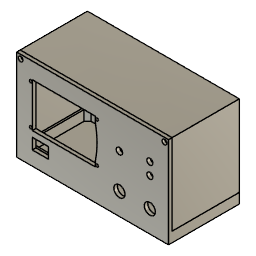
Andrew Block 1 v1 v24 (Autodesk Fusion 360 design; units mm, degrees)
Autodesk Fusion 360 part; units mm, degrees
sketch "Sketch1" plane through (0, 0, 0) normal (0, 0, 1) x (1, 0, 0)
  line L0 (0, 0) -> (190.5, 0)
  line L1 (190.5, 0) -> (190.5, 88.9)
  line L2 (190.5, 88.9) -> (0, 88.9)
  line L3 (0, 88.9) -> (0, 0)
  constraint horizontal L0
  constraint vertical L1
  constraint horizontal L2
  constraint vertical L3
  constraint coincident L0.start L3.end
extrude "Extrude1" add sketch "Sketch1" along normal blind 114.3 makes body 1
ref_plane "WorkPlane1" through (0, 0, 12.7) normal (0, 0, 1) x (1, 0, 0)
shell "Shell1" thickness 4.445 removed faces 0 bodies 1
chamfer "Chamfer4" distance 6.35 angle 45 4 edges at (4.445, 84.455, 57.15) (186.055, 84.455, 57.15) (4.445, 4.445, 57.15) (186.055, 4.445, 57.15) on bodies 1
split "Split1" by plane through (0, 0, 12.7) normal (0, 0, 1) bodies 1 makes body 2 at (127, 88.9, 46.5667)
chamfer "Chamfer5" distance 6.35 angle 45 4 edges at (4.445, 44.45, 109.855) (95.25, 84.455, 109.855) (95.25, 4.445, 109.855) (186.055, 44.45, 109.855) on bodies 2
sketch "Sketch2" plane through (0, 0, 4.445) normal (0, 0, 1) x (-1, 0, 0)
  line L0 (-4.445, -78.105) -> (-4.445, -10.795)
  line L1 (-10.795, -4.445) -> (-179.705, -4.445)
  line L2 (-186.055, -10.795) -> (-186.055, -78.105)
  line L3 (-179.705, -84.455) -> (-10.795, -84.455)
  line L4 (-7.62, -81.28) -> (-182.88, -81.28)
  line L5 (-182.88, -81.28) -> (-182.88, -7.62)
  line L6 (-182.88, -7.62) -> (-7.62, -7.62)
  line L7 (-7.62, -7.62) -> (-7.62, -81.28)
  line L8 (-182.88, -81.28) -> (-184.658, -83.058) construction
  line L9 (-182.88, -81.28) -> (-180.3655, -81.28) construction
  line L10 (-7.62, -7.62) -> (-5.8419, -5.8419) construction
  line L11 (-7.62, -7.62) -> (-5.1054, -7.62) construction
  line L12 (-184.658, -83.058) -> (-5.8419, -83.058)
  line L13 (-5.8419, -83.058) -> (-5.8419, -5.8419)
  line L14 (-5.8419, -5.8419) -> (-184.658, -5.8419)
  line L15 (-184.658, -5.8419) -> (-184.658, -83.058)
  line L16 (-179.705, -4.445) -> (-186.055, -10.795)
  line L17 (-186.055, -78.105) -> (-179.705, -84.455)
  line L18 (-10.795, -84.455) -> (-4.445, -78.105)
  line L19 (-4.445, -10.795) -> (-10.795, -4.445)
  dimension "d7" = 135
  dimension "d8" = 45
  dimension "d9" = 2.5146
  constraint horizontal L4
  constraint vertical L5
  constraint horizontal L6
  constraint vertical L7
  constraint horizontal L9
  constraint horizontal L11
  constraint horizontal L12
  constraint vertical L13
  constraint horizontal L14
  constraint vertical L15
  measures "d7" angle of L8 L9
  measures "d8" angle of L10 L11
  measures "d9" distance of L6.end L10.end
sketch "Sketch6" plane through (0, 0, 0) normal (0, 0, -1) x (1, 0, 0)
  line L0 (0, 0) -> (0, -88.9)
  line L1 (0, -88.9) -> (190.5, -88.9)
  line L2 (190.5, -88.9) -> (190.5, 0)
  line L3 (190.5, 0) -> (0, 0)
  line L4 (5.08, -83.82) -> (185.42, -83.82)
  line L5 (185.42, -83.82) -> (185.42, -5.08)
  line L6 (185.42, -5.08) -> (5.08, -5.08)
  line L7 (5.08, -5.08) -> (5.08, -83.82)
  dimension "d42" = -5.08
sketch "Sketch8" plane through (0, 0, 0) normal (0, -1, 0) x (1, 0, 0)
  line L0 (0, 12.7) -> (190.5, 12.7)
  line L1 (190.5, 12.7) -> (190.5, 114.3)
  line L2 (190.5, 114.3) -> (0, 114.3)
  line L3 (0, 114.3) -> (0, 12.7)
  line L4 (5.08, 17.78) -> (185.42, 17.78)
  line L5 (185.42, 17.78) -> (185.42, 109.22)
  line L6 (185.42, 109.22) -> (5.08, 109.22)
  line L7 (5.08, 109.22) -> (5.08, 17.78)
  dimension "d76" = -5.08
hole "Hole4" at (5.08, 0, 109.22) at (185.42, 0, 109.22) direction (0, 1, 0) diameter 2.54 depth 25.4 tip angle 118 counterbore diameter 5.969 counterbore depth 3.3528 bodies 2
hole "Hole2" at (5.08, 83.82, 0) at (185.42, 83.82, 0) direction (0, 0, 1) diameter 4.318 depth 19.7 tip angle 180 bodies 2
hole "Hole1" at (5.08, 83.82, 0) at (185.42, 83.82, 0) direction (0, 0, 1) diameter 3.556 depth 254 tip angle 118 counterbore diameter 5.969 counterbore depth 3.3528 bodies 1
sketch "Sketch5" plane through (0, 0, 4.445) normal (0, 0, 1) x (-1, 0, 0)
  line L0 (-4.445, -78.105) -> (-4.445, -10.795)
  line L1 (-10.795, -4.445) -> (-179.705, -4.445)
  line L2 (-186.055, -10.795) -> (-186.055, -78.105)
  line L3 (-179.705, -84.455) -> (-10.795, -84.455)
  line L4 (-179.705, -4.445) -> (-186.055, -10.795)
  line L5 (-186.055, -78.105) -> (-179.705, -84.455)
  line L6 (-10.795, -84.455) -> (-4.445, -78.105)
  line L7 (-4.445, -10.795) -> (-10.795, -4.445)
  line L8 (-178.3796, -81.2552) -> (-12.1204, -81.2552)
  line L9 (-12.1204, -81.2552) -> (-7.6448, -76.7796)
  line L10 (-7.6448, -76.7796) -> (-7.6448, -12.1204)
  line L11 (-7.6448, -12.1204) -> (-12.1204, -7.6448)
  line L12 (-12.1204, -7.6448) -> (-178.3796, -7.6448)
  line L13 (-178.3796, -7.6448) -> (-182.8552, -12.1204)
  line L14 (-182.8552, -12.1204) -> (-182.8552, -76.7796)
  line L15 (-182.8552, -76.7796) -> (-178.3796, -81.2552)
  line L16 (-179.3799, -83.6701) -> (-11.1201, -83.6701)
  line L17 (-11.1201, -83.6701) -> (-5.2299, -77.7799)
  line L18 (-5.2299, -77.7799) -> (-5.2299, -11.1201)
  line L19 (-5.2299, -11.1201) -> (-11.1201, -5.2299)
  line L20 (-11.1201, -5.2299) -> (-179.3799, -5.2299)
  line L21 (-179.3799, -5.2299) -> (-185.2701, -11.1201)
  line L22 (-185.2701, -11.1201) -> (-185.2701, -77.7799)
  line L23 (-185.2701, -77.7799) -> (-179.3799, -83.6701)
  dimension "d35" = -3.1998
  dimension "d36" = -0.7849
extrude "Extrude6" add sketch "Sketch5" along normal blind 12.7 contours L16 L17 L18 L19 L20 L21 L22 L23 bodies 1
extrude "Extrude7" add 1 faces at (67.2067, 84.1934, 4.445) along direction (0, 0, 1) blind 5.08 on bodies 1 bodies 1
sketch "Sketch4" plane through (0, 0, 0) normal (0, -1, 0) x (1, 0, 0)
  line L0 (0, 12.7) -> (190.5, 12.7)
  line L1 (190.5, 12.7) -> (190.5, 114.3)
  line L2 (190.5, 114.3) -> (0, 114.3)
  line L3 (0, 114.3) -> (0, 12.7)
  circle A0 centre (128.9671, 27.5835) radius 7
  circle A1 centre (167.0671, 27.5835) radius 7
  circle A2 centre (5.08, 109.22) radius 2.9845
  circle A3 centre (185.42, 109.22) radius 2.9845
  circle A4 centre (167.0671, 78.74) radius 3.81
  circle A5 centre (167.0671, 63.5) radius 3.81
  line L4 (167.0671, 27.5835) -> (167.0671, 63.5) construction
  line L5 (128.9671, 27.5835) -> (128.9671, 63.5) construction
  line L6 (19.812, 17.78) -> (39.878, 17.78)
  line L7 (39.878, 17.78) -> (39.878, 31.496)
  line L8 (19.812, 31.496) -> (19.812, 17.78)
  circle A6 centre (128.9022, 71.12) radius 4.064
  line L9 (15.24, 93.98) -> (103.378, 93.98)
  line L10 (103.378, 93.98) -> (103.378, 38.862)
  line L11 (103.378, 38.862) -> (15.24, 38.862)
  line L12 (15.24, 38.862) -> (15.24, 93.98)
  line L13 (15.24, 93.98) -> (19.812, 93.98)
  line L14 (103.378, 93.98) -> (98.806, 93.98)
  line L15 (19.812, 93.98) -> (19.812, 38.862)
  line L16 (98.806, 93.98) -> (98.806, 38.862)
  line L17 (17.78, 91.44) -> (100.838, 91.44) construction
  line L18 (100.838, 91.44) -> (100.838, 41.402) construction
  line L19 (100.838, 41.402) -> (17.78, 41.402) construction
  line L20 (17.78, 41.402) -> (17.78, 91.44) construction
  line L21 (98.806, 86.4684) -> (100.838, 86.4684)
  line L22 (100.838, 86.4684) -> (100.838, 45.589)
  line L23 (100.838, 45.589) -> (98.806, 45.589)
  line L24 (98.806, 45.589) -> (98.806, 86.4684)
  line L25 (19.812, 31.496) -> (39.878, 31.496)
  line L26 (19.812, 48.3189) -> (19.812, 17.78) construction
  point P0 (128.9671, 63.5)
  dimension "d62" = 14
  dimension "d63" = 14
  dimension "d94" = 7.62
  dimension "d95" = 7.62
  dimension "d103" = 20.066
  dimension "d104" = 13.716
  dimension "d111" = 8.128
  dimension "d114" = 88.138
  dimension "d115" = 55.118
  dimension "d116" = 4.572
  dimension "d117" = 4.572
  dimension "d118" = 2.54
  constraint coincident A1.centre L4.start
  constraint vertical L4
  constraint coincident A0.centre L5.start
  constraint perpendicular L0 L5
  constraint horizontal L6
  constraint vertical L7
  constraint vertical L8
  constraint horizontal L9
  constraint vertical L10
  constraint horizontal L11
  constraint vertical L12
  constraint perpendicular L10 L14
  constraint coincident L11 L15.end
  constraint perpendicular L11 L15
  constraint coincident L11 L16.end
  constraint perpendicular L11 L16
  constraint horizontal L21
  constraint vertical L22
  constraint horizontal L23
  constraint vertical L24
  constraint coincident L18 L22.end
  constraint coincident L16 L21.start
  constraint perpendicular L7 L25
  constraint coincident L15 L26.start
  constraint perpendicular L11 L26
  measures "d62" diameter of A0
  measures "d63" diameter of A1
  measures "d94" diameter of A4
  measures "d95" diameter of A5
  measures "d103" distance of L6.start L6.end
  measures "d104" distance of L6.start L8.start
  measures "d111" diameter of A6
  measures "d114" distance of L9.start L9.end
  measures "d115" distance of L9.start L11.end
  measures "d116" distance of L9.start L13.end
  measures "d117" distance of L9.end L14.end
hole "Hole3" at (17.78, 0, 91.44) at (17.78, 0, 41.402) at (100.838, 0, 91.44) at (100.838, 0, 41.402) direction (0, 1, 0) diameter 3.5 depth 12.7 tip angle 180 bodies 2
extrude "Extrude8" cut sketch "Sketch4" against normal blind 30.48 contours A0 | A1 | A4 | A5 | L6 L7 L8 L25 | A6 | L9 L11 L15 L16 L24 | L16 L21 L22 L23 L24 bodies 2
sketch "Sketch7" plane through (0, 0, 4.445) normal (0, 0, 1) x (-1, 0, 0)
  line L0 (-178.3796, -81.2552) -> (-12.1204, -81.2552)
  line L1 (-7.6448, -76.7796) -> (-7.6448, -12.1204)
  line L2 (-12.1204, -7.6448) -> (-178.3796, -7.6448)
  line L3 (-182.8552, -12.1204) -> (-182.8552, -76.7796)
  line L4 (-76.4252, -76.6519) -> (-76.4252, -12.2481) construction
  circle A0 centre (-76.4252, -76.6519) radius 4.6032
  circle A1 centre (-76.4252, -76.6519) radius 2.159
  circle A2 centre (-76.4252, -12.2481) radius 2.159
  circle A3 centre (-76.4252, -12.2481) radius 4.6032
  line L5 (-12.1204, -81.2552) -> (-7.6448, -76.7796)
  line L6 (-7.6448, -12.1204) -> (-12.1204, -7.6448)
  line L7 (-178.3796, -7.6448) -> (-182.8552, -12.1204)
  line L8 (-182.8552, -76.7796) -> (-178.3796, -81.2552)
  line L9 (-14.0271, -12.2481) -> (-176.4729, -12.2481) construction
  line L10 (-176.4729, -12.2481) -> (-178.2519, -14.0271)
  line L11 (-178.2519, -14.0271) -> (-178.2519, -74.8729) construction
  line L12 (-178.2519, -74.8729) -> (-176.4729, -76.6519)
  line L13 (-176.4729, -76.6519) -> (-14.0271, -76.6519) construction
  line L14 (-14.0271, -76.6519) -> (-12.2481, -74.8729)
  line L15 (-12.2481, -74.8729) -> (-12.2481, -14.0271) construction
  line L16 (-12.2481, -14.0271) -> (-14.0271, -12.2481)
  line L17 (-162.5137, -12.2481) -> (-162.5137, -76.6519) construction
  circle A4 centre (-162.7852, -12.8831) radius 4.6032
  circle A5 centre (-162.7852, -12.8831) radius 2.159
  circle A6 centre (-162.7852, -76.0169) radius 4.6032
  circle A7 centre (-162.7852, -76.0169) radius 2.159
  dimension "d52" = -4.6032
  dimension "d53" = 4.318
  dimension "d56" = 4.318
  dimension "d71" = 4.318
  dimension "d72" = 4.318
  constraint coincident L4.start L13
  constraint coincident L4.end L9
  constraint perpendicular L4 L9
  constraint coincident L4.start A0.centre
  constraint tangent L0 A0
  constraint concentric A0 A1
  constraint concentric A2 A3
  constraint tangent L2 A3
  constraint coincident L9 L17.start
  constraint coincident L13 L17.end
  constraint perpendicular L13 L17
  constraint concentric A4 A5
  constraint concentric A6 A7
  measures "d53" diameter of A1
  measures "d56" diameter of A2
  measures "d71" diameter of A5
  measures "d72" diameter of A7
ref_plane "WorkPlane2" through (0, 4.445, 0) normal (0, 1, 0) x (0, 0, 1)
chamfer "Chamfer3" distance 1.016 angle 45 1 edges at (187.4329, 84.6007, 12.7) on bodies 2
chamfer "Chamfer3" distance 1.016 angle 45 1 edges at (7.0929, 84.6007, 12.7) on bodies 2
split "Split2" by plane through (0, 4.445, 0) normal (0, 1, 0) bodies 2 makes body 3 at (127, 88.9, 46.5667)
fillet "Fillet1" radius 99.06 2 edges at (100.838, 2.2225, 86.4684) (100.838, 2.2225, 45.589) on bodies 2
combine "Combine1" operation add target body 1 tool bodies 2
hole "Hole5" at (5.08, 0, 109.22) at (185.42, 0, 109.22) direction (0, 1, 0) diameter 4.318 depth 19.7 tip angle 180 bodies 3
sketch "Sketch11" plane through (0, 4.445, 0) normal (0, 1, 0) x (-1, 0, 0)
  circle A0 centre (-167.0671, 27.5835) radius 7
  circle A1 centre (-167.0671, 78.74) radius 3.81
  circle A2 centre (-128.9671, 27.5835) radius 7
  circle A3 centre (-167.0671, 63.5) radius 3.81
  circle A4 centre (-5.08, 109.22) radius 1.27
  circle A5 centre (-185.42, 109.22) radius 1.27
  line L0 (-179.705, 9.525) -> (-10.795, 9.525)
  line L1 (-10.795, 9.525) -> (-10.795, 12.7)
  line L2 (-10.795, 12.7) -> (0, 12.7)
  line L3 (0, 12.7) -> (0, 114.3)
  line L4 (0, 114.3) -> (-190.5, 114.3)
  line L5 (-190.5, 114.3) -> (-190.5, 12.7)
  line L6 (-190.5, 12.7) -> (-179.705, 12.7)
  line L7 (-179.705, 12.7) -> (-179.705, 9.525)
  circle A6 centre (-128.9022, 71.12) radius 4.064
  circle A7 centre (-100.838, 41.402) radius 1.75
  circle A8 centre (-17.78, 41.402) radius 1.75
  circle A9 centre (-17.78, 91.44) radius 1.75
  circle A10 centre (-100.838, 91.44) radius 1.75
  line L8 (-19.812, 38.862) -> (-98.806, 38.862)
  line L9 (-98.806, 38.862) -> (-98.806, 45.589)
  arc A11 (-100.838, 65.5503) -> (-98.806, 45.589) centre (-1.778, 65.5503) ccw
  line L10 (-100.838, 65.5503) -> (-100.838, 66.5072)
  arc A12 (-98.806, 86.4684) -> (-100.838, 66.5072) centre (-1.778, 66.5072) ccw
  line L11 (-98.806, 86.4684) -> (-98.806, 93.98)
  line L12 (-98.806, 93.98) -> (-19.812, 93.98)
  line L13 (-19.812, 93.98) -> (-19.812, 38.862)
  line L14 (-39.878, 17.78) -> (-39.878, 31.496)
  line L15 (-39.878, 31.496) -> (-19.812, 31.496)
  line L16 (-19.812, 31.496) -> (-19.812, 17.78)
  line L17 (-19.812, 17.78) -> (-39.878, 17.78)
sketch "Sketch12" plane through (0, 0, 4.445) normal (0, 0, 1) x (-1, 0, 0)
  line L0 (-170.18, -83.6676) -> (-106.68, -83.6676)
  line L1 (-106.68, -83.6676) -> (-106.68, -78.5876)
  line L2 (-106.68, -78.5876) -> (-170.18, -78.5876)
  line L3 (-170.18, -78.5876) -> (-170.18, -83.6676)
  dimension "d107" = 63.5
  constraint horizontal L0
  constraint vertical L1
  constraint horizontal L2
  constraint vertical L3
  measures "d107" distance of L1.end L2.end
extrude "Extrude11" add sketch "Sketch12" along normal blind 66.04 bodies 1
chamfer "Chamfer6" distance 1.016 angle 45 2 edges at (186.2007, 4.445, 111.2329) (5.8607, 4.445, 111.2329) on bodies 3
move_body "Move3" [suppressed]
sketch "Sketch9" plane through (0, 0, 4.445) normal (0, 0, 1) x (-1, 0, 0)
  line L0 (-178.3796, -81.2552) -> (-12.1204, -81.2552)
  line L1 (-12.1204, -81.2552) -> (-7.6448, -76.7796)
  line L2 (-7.6448, -76.7796) -> (-7.6448, -12.1204)
  line L3 (-7.6448, -12.1204) -> (-12.1204, -7.6448)
  line L4 (-12.1204, -7.6448) -> (-178.3796, -7.6448)
  line L5 (-178.3796, -7.6448) -> (-182.8552, -12.1204)
  line L6 (-182.8552, -12.1204) -> (-182.8552, -76.7796)
  line L7 (-182.8552, -76.7796) -> (-178.3796, -81.2552)
  line L8 (-106.68, -68.58) -> (-25.4, -68.58)
  line L9 (-25.4, -68.58) -> (-25.4, -17.78)
  line L10 (-25.4, -17.78) -> (-106.68, -17.78)
  line L11 (-106.68, -17.78) -> (-106.68, -68.58)
  line L12 (-106.68, -68.58) -> (-25.4, -17.78) construction
  line L13 (-25.4, -68.58) -> (-106.68, -17.78) construction
  point P0 (-66.04, -43.18)
  dimension "d86" = 81.28
  dimension "d87" = 50.8
  constraint horizontal L8
  constraint perpendicular L8 L9
  constraint parallel L8 L10
  constraint parallel L9 L11
  constraint coincident L12 P0
  constraint coincident L13 P0
  measures "d86" distance of L9.end L10.end
  measures "d87" distance of L8.end L9.end
equation "d32 = 7 mm + 0.5 in"
equation "d82 = 7 mm + 0.5 in"
